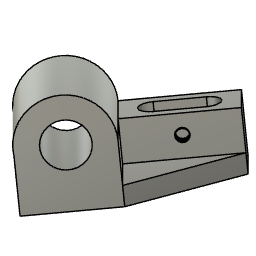
design1 (Autodesk Fusion 360 design; units mm, degrees)
Autodesk Fusion 360 part; units mm, degrees
sketch "Sketch1" plane through (0, 0, 0) normal (1, 0, 0) x (0, 1, 0)
sketch "Sketch1 (2)" plane through (0, 0, 0) normal (0, 0, 1) x (1, 0, 0) in component "Box"
  line L0 (-20.9827, 18.7375) -> (142.0173, 18.7375)
  line L1 (142.0173, 18.7375) -> (142.0173, -31.2625)
  line L2 (142.0173, -31.2625) -> (-20.9827, -31.2625)
  line L3 (-20.9827, -31.2625) -> (-20.9827, 18.7375)
  circle A0 centre (104.8115, 18.7375) radius 37.5
  line L4 (142.0173, 18.7375) -> (104.5173, 18.7375)
  line L5 (104.8115, 18.7375) -> (100, 18.7375)
  circle A1 centre (104.5173, 18.7375) radius 18.75
  line L6 (-20.9827, 18.7375) -> (67.0173, 18.7375)
  line L7 (67.0173, 18.7375) -> (67.0173, -15.2625)
  line L8 (67.0173, -15.2625) -> (-20.9827, -15.2625)
  line L9 (-20.9827, -15.2625) -> (-20.9827, 18.7375)
  dimension "d1" = 163
  dimension "d2" = 50
  dimension "d3" = 75
  dimension "d4" = 37.5
  dimension "d5" = 37.5
  dimension "d6" = 88
  dimension "d7" = 34
  constraint horizontal L0
  constraint vertical L1
  constraint horizontal L2
  constraint vertical L3
  constraint coincident L0 A0.centre
  constraint perpendicular L1 L4
  constraint coincident A0.centre L5.start
  constraint coincident L0 L5.end
  constraint perpendicular L1 L5
  constraint coincident L4.end A1.centre
  constraint horizontal L6
  constraint vertical L7
  constraint horizontal L8
  constraint vertical L9
  measures "d1" distance of L0.start L0.end
  measures "d2" distance of L0.start L2.end
  measures "d3" diameter of A0
  measures "d4" distance of L0.end L4.end
  measures "d5" diameter of A1
  measures "d6" distance of L0.start L6.end
  measures "d7" distance of L0.start L8.end
sketch "Sketch2" plane through (0, 0, 0) normal (0, 0, 1) x (1, 0, 0) in component "Box"
extrude "Extrude1" add sketch "Sketch1 (2)" along normal blind 88 contours L0 L3 L6 L7 L8 L9 | L0 L1 L2 L3 A0 L7 L8 | L0 L1 A0 L4 A1 | L0 L1 A0 L4 A1 in component "Box"
sketch "Sketch3" plane through (0, 0, 0) normal (0, 0, -1) x (1, 0, 0) in component "Box"
  circle A0 centre (104.5173, -18.7375) radius 18.75
  arc A1 (67.3115, -18.7375) -> (142.0173, -14.0489) centre (104.8115, -18.7375) ccw
  line L0 (142.0173, -14.0489) -> (142.0173, 31.2625)
  line L1 (142.0173, 31.2625) -> (-20.9827, 31.2625)
  line L2 (-20.9827, 31.2625) -> (-20.9827, -18.7375)
  line L3 (-20.9827, -18.7375) -> (67.3115, -18.7375)
sketch "Sketch4" plane through (0, 0, 0) normal (0, 0, -1) x (1, 0, 0) in component "Box"
sketch "Sketch5" plane through (0, 18.7375, 0) normal (0, 1, 0) x (-1, 0, 0) in component "Box"
  line L0 (-67.3115, 0) -> (20.9827, 0)
  line L1 (20.9827, 0) -> (20.9827, 88)
  line L2 (20.9827, 88) -> (-67.3115, 88)
  line L3 (-67.3115, 88) -> (-67.3115, 0)
  line L4 (-67.3115, 88) -> (20.6885, 88)
  line L5 (20.6885, 88) -> (20.6885, 48)
  line L6 (20.6885, 48) -> (-67.3115, 48)
  line L7 (-67.3115, 48) -> (-67.3115, 88)
  line L8 (-42.3115, 57) -> (-4.3115, 57)
  arc A0 (-4.3115, 57) -> (-4.3115, 79) centre (-4.3115, 68) ccw
  line L9 (-4.3115, 79) -> (-42.3115, 79)
  arc A1 (-42.3115, 79) -> (-42.3115, 57) centre (-42.3115, 68) ccw
  line L10 (-42.3115, 68) -> (-4.3115, 68) construction
  line L11 (-42.3115, 68) -> (-56.3288, 68)
  line L12 (-56.3288, 68) -> (-42.3115, 68)
  dimension "d11" = 88
  dimension "d12" = 40
  dimension "d13" = 22
  dimension "d14" = 11
  dimension "d15" = 38
  dimension "d16" = 20
  dimension "d20" = 25
  dimension "d22" = 20
  constraint horizontal L4
  constraint vertical L5
  constraint horizontal L6
  constraint vertical L7
  constraint coincident L2.end L3.start
  constraint tangent L8 A0
  constraint tangent A0 L9
  constraint parallel L8 L9
  constraint tangent L9 A1
  constraint tangent L8 A1
  constraint perpendicular L3 L10
  constraint coincident A1.centre L10.start
  constraint parallel L10 L11
  measures "d11" distance of L2.end L4.end
  measures "d12" distance of L2.end L6.end
  measures "d13" diameter of A0
  measures "d14" radius of A1
  measures "d15" distance of A1.centre A0.centre
  measures "d16" distance of L6 L11.end
  measures "d20" distance of L5 A0.centre
  measures "d22" distance of L4 A0.centre
extrude "Extrude2" cut sketch "Sketch5" against normal blind 34 contours L8 A0 L9 A1 in component "Box"
sketch "Sketch6" plane through (0, 0, 0) normal (0, 0, -1) x (1, 0, 0) in component "Box"
  line L0 (67.0173, 15.2625) -> (-20.9827, 15.2625)
  line L1 (-20.9827, -18.7375) -> (142.0173, -18.7375)
  point P0 (-20.9827, -18.7375)
  dimension "d25" = 88
  measures "d25" distance of L0.start L0.end
sketch "Sketch7" plane through (0, 18.7375, 0) normal (0, 1, 0) x (-1, 0, 0) in component "Box"
  line L0 (-4.3115, 57) -> (-42.3115, 57)
  arc A0 (-42.3115, 79) -> (-42.3115, 57) centre (-42.3115, 68) ccw
  line L1 (-42.3115, 79) -> (-4.3115, 79)
  arc A1 (-4.3115, 57) -> (-4.3115, 79) centre (-4.3115, 68) ccw
  line L2 (-67.3115, 0) -> (20.9827, 0)
  line L3 (20.9827, 0) -> (20.9827, 88)
  line L4 (20.9827, 88) -> (-67.3115, 88)
  line L5 (-67.3115, 88) -> (-67.3115, 0)
  line L6 (-67.3115, 88) -> (20.6885, 88)
  line L7 (20.6885, 88) -> (20.6885, 48)
  line L8 (20.6885, 48) -> (-67.3115, 48)
  line L9 (-67.3115, 48) -> (-67.3115, 88)
  line L10 (-67.3115, 0) -> (20.6885, 48)
  dimension "d26" = 88
  dimension "d27" = 40
  constraint horizontal L6
  constraint vertical L7
  constraint horizontal L8
  constraint vertical L9
  constraint coincident L4.end L5.start
  constraint coincident L2.start L5.end
  measures "d26" distance of L4.end L6.end
  measures "d27" distance of L4.end L8.end
extrude "Extrude3" cut sketch "Sketch7" against normal blind 70 contours L2 L3 L4 L7 L10 in component "Box"
extrude "Extrude4" cut sketch "Sketch5" against normal blind 34 contours L0 L1 L2 L3 L5 L6 in component "Box"
sketch "Sketch8" plane through (0, 0, 0) normal (0, 0, 1) x (1, 0, 0) in component "Box"
  line L0 (-20.6885, 18.7375) -> (67.3115, 18.7375)
  line L1 (67.3115, -15.2625) -> (-20.6885, -15.2625)
  dimension "d32" = 34
  measures "d32" distance of L0 L1
sketch "Sketch9" plane through (0, 0, 0) normal (0, 0, -1) x (1, 0, 0) in component "Box"
sketch "Sketch10" plane through (23.3115, 18.7375, 68) normal (0, 1, 0) x (-1, 0, 0) in component "Box"
sketch "Sketch11" plane through (0, 0, 48) normal (0, 0, -1) x (1, 0, 0) in component "Box"
  line L0 (-20.6885, -18.7375) -> (67.3115, -18.7375)
  line L1 (67.3115, -18.7375) -> (67.3115, 15.2625)
  line L2 (67.3115, 15.2625) -> (-20.6885, 15.2625)
  line L3 (-20.6885, 15.2625) -> (-20.6885, -18.7375)
  circle A0 centre (23.0173, -1.7375) radius 6
  line L4 (-20.9827, 31.2625) -> (-20.9827, -18.7375)
  point P0 (23.3115, -18.7375)
  dimension "d33" = 12
  dimension "d34" = 44
  measures "d33" diameter of A0
  measures "d34" distance of A0.centre L4
extrude "Extrude5" cut sketch "Sketch11" against normal blind 15 contours A0 in component "Box"
thread "Thread1" "ISO Metric profile 12.0 M12x1.75 6H" major diameter 12.2265 minor diameter 10.2735 pitch 1.75 angle 60 modelled right hand crest width 0.4769 on face at (28.9875, 2.3349, 51) crest through (28.154, 1.7375, 48.4375) in component "Box"
sketch "Sketch12" plane through (23.3115, 18.7375, 68) normal (0, 1, 0) x (-1, 0, 0) in component "Box"
sketch "Sketch13" plane through (0, 0, 48) normal (0, 0, -1) x (1, 0, 0) in component "Box"
  line L0 (-20.6885, -18.7375) -> (67.3115, -18.7375)
  line L1 (67.3115, -18.7375) -> (67.3115, 15.2625)
  line L2 (67.3115, 15.2625) -> (-20.6885, 15.2625)
  line L3 (-20.6885, 15.2625) -> (-20.6885, -18.7375)
  spline S0 degree 3 poles (26.8972, 1.6288) (27.3873, 1.1607) (27.7795, 0.5999) (28.3411, -0.6611) (28.4966, -1.3528) (28.539, -2.7813) (28.4163, -3.5045) (27.8961, -4.8878) (27.4951, -5.5312) (26.6594, -6.4302) (26.294, -6.738) (25.4903, -7.2656) (25.0537, -7.4815) (24.5962, -7.6434) knots 0 0 0 0 0.203323 0.203323 0.413794 0.413794 0.631411 0.631411 0.856169 0.856169 0.998571 0.998571 1.143699 1.143699 1.143699 1.143699
  arc A0 (21.4384, -7.6434) -> (24.5962, -7.6434) centre (23.0173, -1.7375) ccw
  spline S1 degree 3 poles (21.4384, -7.6434) (20.7013, -7.3826) (20.0213, -6.9825) (18.8741, -5.957) (18.4119, -5.3483) (17.7613, -4.0077) (17.571, -3.2929) (17.4813, -1.8543) (17.5735, -1.1452) (17.9375, -0.0726) (18.1213, 0.3117) (18.5728, 1.0196) (18.8371, 1.342) (19.1373, 1.6288) knots 0 0 0 0 0.234557 0.234557 0.461953 0.461953 0.682185 0.682185 0.895249 0.895249 1.022941 1.022941 1.14791 1.14791 1.14791 1.14791
  arc A1 (26.8972, 1.6288) -> (19.1373, 1.6288) centre (23.0173, -1.7375) ccw
  circle A2 centre (23.0173, -1.7375) radius 5.137
  dimension "d38" = 10.274
  constraint concentric A0 A2
  measures "d38" diameter of A2
component "Box" placed x (1, 0, 0) y (0, 1, 0) z (0, 0, 1) at (0, 0, 0)
